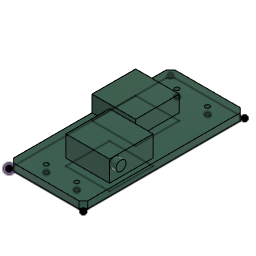
MT3608 Step-up v2 (Autodesk Fusion 360 design; units mm, degrees)
Autodesk Fusion 360 part; units mm, degrees
sketch "Skizze1" plane through (0, 0, 0) normal (0, 0, 1) x (1, 0, 0)
  line L0 (1, 0) -> (16, 0)
  line L1 (17, 1) -> (17, 36)
  line L2 (16, 37) -> (1, 37)
  line L3 (0, 36) -> (0, 1)
  circle A0 centre (5, 33.5) radius 0.5
  circle A1 centre (12, 33.5) radius 0.5
  circle A2 centre (5, 3.5) radius 0.5
  circle A3 centre (12, 3.5) radius 0.5
  line L4 (0, 29) -> (10, 29)
  line L5 (10, 29) -> (10, 19)
  line L6 (10, 19) -> (0, 19)
  line L7 (0, 19) -> (0, 29)
  line L8 (16, 7) -> (6, 7)
  line L9 (6, 7) -> (6, 17)
  line L10 (6, 17) -> (16, 17)
  line L11 (16, 17) -> (16, 7)
  line L12 (1, 37) -> (0, 36)
  line L13 (17, 36) -> (16, 37)
  line L14 (1, 0) -> (0, 1)
  line L15 (16, 0) -> (17, 1)
  point P0 (17, 0)
  point P1 (17, 37)
  point P2 (0, 37)
  dimension "d1" = 17
  dimension "d2" = 37
  dimension "d3" = 1
  dimension "d4" = 5
  dimension "d5" = 3.5
  dimension "d8" = 7
  dimension "d9" = -30
  dimension "d10" = 10
  dimension "d11" = 10
  dimension "d12" = 8
  dimension "d13" = 10
  dimension "d14" = 10
  dimension "d15" = 7
  dimension "d16" = 1
  dimension "d28" = 1
  dimension "d29" = 1
  dimension "d30" = 1
  dimension "d31" = 1
  dimension "d32" = 1
  dimension "d33" = 1
  dimension "d34" = 1
  dimension "d35" = 1
  constraint horizontal L0
  constraint vertical L1
  constraint horizontal L2
  constraint vertical L3
  constraint horizontal L4
  constraint vertical L5
  constraint horizontal L6
  constraint vertical L7
  constraint coincident L3 L4.start
  constraint horizontal L8
  constraint vertical L9
  constraint horizontal L10
  constraint vertical L11
  constraint coincident P2 L2
  constraint coincident P2 L3
  constraint coincident P1 L1
  constraint coincident P1 L2
  constraint coincident origin L0
  constraint coincident origin L3
  constraint coincident P0 L0
  constraint coincident P0 L1
  measures "d1" distance of origin P0
  measures "d2" distance of origin P2
  measures "d3" diameter of A0
  measures "d4" distance of L3 A0.centre
  measures "d5" distance of L2 A0.centre
  measures "d10" distance of L4.start L4.end
  measures "d11" distance of L4.start L6.end
  measures "d12" distance of L2 L4
  measures "d13" distance of L8.start L8.end
  measures "d14" distance of L8.start L10.end
  measures "d15" distance of L0 L8
  measures "d16" distance of L1 L11
  measures "d28" distance of P2 L2.end
  measures "d29" distance of P2 L3.start
  measures "d30" distance of P1 L1.end
  measures "d31" distance of P1 L2.start
  measures "d32" distance of origin L0.start
  measures "d33" distance of origin L3.end
  measures "d34" distance of P0 L0.end
  measures "d35" distance of P0 L1.start
extrude "Extrusion1" add sketch "Skizze1" along normal blind 1.6 contours L0 L1 L2 L3 L4 L5 L6 L12 L13 L14 L15
extrude "Extrusion2" add sketch "Skizze1" along normal blind 5.3 contours L3 L4 L5 L6 L7
extrude "Extrusion3" add sketch "Skizze1" along normal blind 6.4 contours L8 L9 L10 L11
sketch "Skizze2" plane through (16, 0, 0) normal (1, 0, 0) x (0, 1, 0)
  line L0 (17, 1.6) -> (17, 6.4)
  line L1 (17, 6.4) -> (7, 6.4)
  line L2 (7, 6.4) -> (7, 1.6)
  circle A0 centre (8.15, 5.25) radius 1.15
  line L3 (7, 1.6) -> (17, 1.6)
  dimension "d23" = 2.3
  dimension "d24" = 1.15
  dimension "d25" = 1.15
  measures "d23" diameter of A0
  measures "d24" distance of L2 A0.centre
  measures "d25" distance of L1 A0.centre
extrude "Extrusion4" add sketch "Skizze2" along normal blind 1.5 contours A0
equation "d29 = d28"
equation "d31 = d30"
equation "d33 = d32"
equation "d35 = d34"
